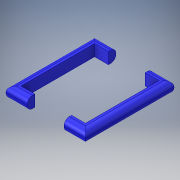
# Autodesk Inventor part: Bumbers.ver1-1111-2019
Saved by Autodesk Inventor 2018 (Build 220112000, 112)
## iProperties
Created: 2020-01-06
Part Number: Bumbers.ver1-1111-2019
Material: Nylon 6/6
Document SubType Name: Modeling
Designer: JMHal
Density: 1.13 g/cm^3
Appearance: Nylon 6
Author: JMHal
Autodesk Inventor part; units mm, degrees
ref_plane "YZ Plane" through (0, 0, 0) normal (1, 0, 0) x (0, 1, 0)
ref_plane "XZ Plane" through (0, 0, 0) normal (0, 1, 0) x (-1, 0, 0)
ref_plane "XY Plane" through (0, 0, 0) normal (0, 0, 1) x (1, 0, 0)
sketch "Sketch1" plane through (0, 0, 0) normal (0, 1, 0) x (-1, 0, 0)
  line L0 (0, 0) -> (711.2, 0)
  line L1 (711.2, 0) -> (711.2, -812.8)
  line L2 (711.2, -812.8) -> (0, -812.8)
  line L3 (0, -812.8) -> (0, 0)
  line L4 (793.75, -895.35) -> (793.75, 82.55)
  line L5 (793.75, 82.55) -> (-82.55, 82.55)
  line L6 (-82.55, 82.55) -> (-82.55, -895.35)
  line L7 (-82.55, -895.35) -> (793.75, -895.35)
  dimension "d0" = 812.8
  dimension "d1" = 711.2
  dimension "d2" = 82.55
  constraints: 16 end point, 4 parallel, 2 perpendicular, 1 horizontal, 3 other
  measures "d0" distance of L0.end L1.end
  measures "d1" distance of L1.end L2.end
  measures "d2" distance between parallel lines of L1 L4
extrude "Extrusion1" add sketch "Sketch1" along normal blind 127
fillet "Fillet1" radius 57.15 8 edges at (82.55, 127, -406.4) (82.55, 0, -406.4) (-355.6, 0, 82.55) (-355.6, 127, 82.55) (-355.6, 127, -895.35) (-355.6, 0, -895.35) (-793.75, 127, -406.4) (-793.75, 0, -406.4)
sketch "Sketch2" plane through (0, 0, 0) normal (0, 0, -1) x (-1, 0, 0)
  line L0 (711.2, 0) -> (0, 0) projected
  line L1 (711.2, 0) -> (711.2, 127) projected
  line L2 (0, 127) -> (711.2, 127) projected
  line L3 (0, 0) -> (0, 127) projected
  line L4 (558.8, 127) -> (558.8, 0)
  line L5 (711.2, 0) -> (0, 0) projected
  line L6 (0, 127) -> (711.2, 127) projected
  line L7 (152.4, 127) -> (152.4, 0)
  line L8 (355.6, 0) -> (355.6, 127)
  dimension "d6" = 406.4
  constraints: 6 end point, 4 point on line, 2 midpoint, 1 perpendicular, 1 vertical, 1 other
  measures "d6" distance between parallel lines of L4 L7
extrude "Extrusion2" cut sketch "Sketch2" against normal blind 127 contours L0 L8 L2 L4 | L0 L7 L2 L8
ref_plane "Work Plane1" through (-793.75, 57.15, -406.4) normal (0, 0, 1) x (1, 0, 0)
mirror "Mirror1" about plane through (-793.75, 57.15, -406.4) normal (0, 0, 1) of "Extrusion2"
body "Solid1"
